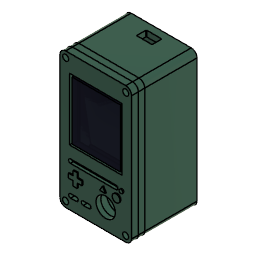
BMO (Autodesk Fusion 360 design; units mm, degrees)
Autodesk Fusion 360 part; units mm, degrees
note: some values were not read from the file. Chosen so that the rebuilt part matches the saved one: which bodies a step acts on; which face or edge a step refers to.
sketch "Sketch1" plane through (0, 0, 0) normal (0, 0, 1) x (1, 0, 0)
  line L0 (-25, -20) -> (2, -20)
  line L1 (2, -20) -> (2, 20)
  line L2 (2, 20) -> (-25, 20)
  line L3 (-25, 20) -> (-25, -20)
  dimension "d1" = 27
  dimension "d2" = 40
  constraint horizontal L0
  constraint vertical L1
  constraint horizontal L2
  constraint vertical L3
  measures "d1" distance of L0.start L0.end
  measures "d2" distance of L0.start L2.end
extrude "Extrude1" add sketch "Sketch1" along normal blind 2 makes body 1
sketch "Sketch2" plane through (0, 0, 2) normal (0, 0, 1) x (-1, 0, 0)
  line L0 (25, -20) -> (25, 20)
  line L1 (25, 20) -> (-2, 20)
  line L2 (-2, 20) -> (-2, -20)
  line L3 (-2, -20) -> (25, -20)
  line L4 (11.5, 20) -> (11.5, 16)
  line L5 (11.5, -20) -> (11.5, -15)
  line L6 (25, -15) -> (-2, -15)
  line L7 (-2, -15) -> (-2, 15)
  line L8 (25, 15) -> (25, -15)
  line L9 (25, 15) -> (-2, 15)
  dimension "d5" = 4
  dimension "d6" = 5
  constraint midpoint L1 L4.start
  constraint perpendicular L1 L4
  constraint midpoint L3 L5.start
  constraint perpendicular L3 L5
  constraint coincident L0 L6.start
  constraint coincident L2 L6.end
  constraint perpendicular L2 L6
  constraint coincident L2 L7.end
  constraint perpendicular L1 L7
  constraint coincident L0 L8.start
  constraint perpendicular L7 L9
  measures "d5" distance of L4.start L4.end
  measures "d6" distance of L5.start L5.end
extrude "Extrude2" add sketch "Sketch2" along normal blind 3 contours L0 L2 L6 L7 L8 L9 bodies 1
sketch "Sketch3" plane through (0, 0, 5) normal (0, 0, 1) x (-1, 0, 0)
  line L0 (25, -15) -> (25, 15)
  line L1 (25, 15) -> (-2, 15)
  line L2 (-2, 15) -> (-2, -15)
  line L3 (-2, -15) -> (25, -15)
  line L4 (-1, 15) -> (-1, -15)
  line L5 (24, -15) -> (24, 15)
  dimension "d9" = -1
  dimension "d10" = -1
extrude "Extrude3" cut sketch "Sketch3" against normal up to surface (3 mm away) contours L1 L2 L3 L4 bodies 1
extrude "Extrude4" cut sketch "Sketch3" against normal up to surface (3 mm away) contours L0 L1 L3 L5 bodies 1
sketch "Sketch4" plane through (0, 0, 0) normal (0, 0, 1) x (1, 0, 0)
  line L0 (-5, -8) -> (22, -8)
  line L1 (22, -8) -> (22, 22)
  line L2 (22, 22) -> (-5, 22)
  line L3 (-5, 22) -> (-5, -8)
  line L4 (27, -13) -> (27, 27)
  line L5 (27, 27) -> (-10, 27)
  line L6 (-10, 27) -> (-10, -13)
  line L7 (-5, -13) -> (22, -13)
  line L8 (-10, -13) -> (-10, -38)
  line L9 (27, -13) -> (27, -38)
  line L10 (-10, -38) -> (-5, -38)
  line L11 (27, -38) -> (22, -38)
  line L12 (-5, -38) -> (-5, -13)
  line L13 (22, -38) -> (22, -13)
  dimension "d15" = 27
  dimension "d16" = 30
  dimension "d18" = 25
  dimension "d19" = 25
  dimension "d20" = 5
  dimension "d21" = 5
  constraint horizontal L0
  constraint vertical L1
  constraint horizontal L2
  constraint vertical L3
  constraint perpendicular L7 L8
  constraint perpendicular L7 L9
  constraint perpendicular L8 L10
  constraint perpendicular L9 L11
  constraint perpendicular L7 L12
  constraint perpendicular L7 L13
  measures "d15" distance of L0.start L0.end
  measures "d16" distance of L0.start L2.end
  measures "d18" distance of L6.end L8.end
  measures "d19" distance of L4.start L9.end
  measures "d20" distance of L8.end L10.end
  measures "d21" distance of L9.end L11.end
extrude "Extrude5" add sketch "Sketch4" along normal blind 5 separate body makes body 2
move_body "Move1" bodies 2 to x (1, 0, 0) y (0, 1, 0) z (0, 0, 1) at (-20, -7, -1)
extrude "Extrude6" cut 1 faces at (-7, 15, 2.3333) along direction (0, 1, 0) blind 1 on bodies 2 bodies 2
extrude "Extrude7" cut 1 faces at (-16, -15, 2.3333) along direction (0, -1, 0) blind 1 on bodies 2 bodies 2
sketch "Sketch5" plane through (0, -20, 0) normal (0, -1, 0) x (1, 0, 0)
  line L0 (-25, -1) -> (2, -1)
  line L1 (2, -1) -> (2, 4)
  line L2 (2, 4) -> (-25, 4)
  line L3 (-25, 4) -> (-25, -1)
  line L4 (-11.5, 0.2) -> (2, 0.2)
  line L5 (-11.5, 0.2) -> (-25, 0.2)
  line L6 (-25, 0.2) -> (-25, 1.4)
  line L7 (-25, 1.4) -> (2, 1.5)
  line L8 (2, 0.2) -> (2, 1.5)
  dimension "d29" = 1.2
  constraint coincident L1 L4.end
  constraint perpendicular L1 L4
  constraint coincident L3 L5.end
  constraint perpendicular L3 L5
  constraint perpendicular L5 L6
  constraint midpoint L1 L7.end
  measures "d29" distance of L5.end L6.end
extrude "Extrude8" cut sketch "Sketch5" against normal blind 42 contours L1 L3 L4 L5 L6 L7 L8 bodies 2
extrude "Extrude9" add 1 faces at (5.3333, -13.6667, 4) along direction (0, 0, 1) blind 2 on bodies 2 bodies 2
sketch "Sketch6" plane through (0, 20, 0) normal (0, 1, 0) x (-1, 0, 0)
  line L0 (-2, 0.2) -> (-2, 1.5)
  line L1 (-2, 1.5) -> (25, 1.4)
  line L2 (25, 1.4) -> (25, 0.2)
  line L3 (25, 0.2) -> (-2, 0.2)
  line L4 (-7, -1) -> (30, -1)
  line L5 (30, -1) -> (30, 6)
  line L6 (30, 6) -> (-7, 6)
  line L7 (-7, 6) -> (-7, -1)
  line L8 (-2, 0) -> (-2.5, 0)
  line L9 (-2.5, 2) -> (-2, 2)
  line L10 (25, 2) -> (25.5, 2)
  line L11 (25.5, 0) -> (-2, 0)
  line L12 (-2, 2) -> (-1, 2)
  line L13 (-1, 2) -> (-1, 5.2)
  line L14 (25, 2) -> (24, 2)
  line L15 (24, 2) -> (24, 5.2)
  line L16 (24, 5.2) -> (-1, 5.2)
  line L17 (25.5, 2) -> (25.5, 0)
  line L18 (-2.5, 0) -> (-2.5, 2)
  dimension "d36" = 1
  dimension "d38" = 1
  dimension "d39" = 3.2
  constraint perpendicular L0 L8
  constraint perpendicular L2 L10
  constraint perpendicular L13 L16
  measures "d36" distance of L9.end L12.end
  measures "d38" distance of L10.start L14.end
  measures "d39" distance of L14.end L15.end
extrude "Extrude10" cut sketch "Sketch6" against normal blind 40.5 contours L8 L9 L10 L11 L12 L13 L14 L15 L16 L17 L18 bodies 2
move_body "Move2" bodies 2 to x (1, 0, 0) y (0, 0, 1) z (0, -1, 0) at (0, -42.5, 47.5)
sketch "Sketch7" plane through (0, 0, 0) normal (0, 0, 1) x (1, 0, 0)
  line L0 (2, 41) -> (-25, 41)
  line L1 (7, 46) -> (-30, 46)
  line L2 (7, 46) -> (7, -29)
  line L3 (2, 41) -> (2, -29)
  line L4 (-25, 41) -> (-25, -29)
  line L5 (-30, 46) -> (-30, -29)
  line L6 (7, -29) -> (2, -29)
  line L7 (-25, -29) -> (-30, -29)
  dimension "d58" = 75
  dimension "d59" = 70
  dimension "d60" = 70
  dimension "d61" = 75
  constraint perpendicular L1 L2
  constraint perpendicular L0 L3
  constraint perpendicular L0 L4
  constraint perpendicular L1 L5
  measures "d58" distance of L1.start L2.end
  measures "d59" distance of L0.start L3.end
  measures "d60" distance of L0.end L4.end
  measures "d61" distance of L1.end L5.end
extrude "Extrude11" add sketch "Sketch7" along normal blind 7 separate body makes body 3
move_body "Move3" bodies 3 to x (1, 0, 0) y (0, 1, 0) z (0, 0, 1) at (0, -12.5, 2.5)
move_body "Move6" bodies 2 to x (1, 0, 0) y (0, 0.866025, -0.5) z (0, 0.5, 0.866025) at (0, -6.2478, -21.317)
move_body "Move7" bodies 1 to x (1, 0, 0) y (0, 0.573576, 0.819152) z (0, -0.819152, 0.573576) at (0, -8.5285, 16.383)
move_body "Move8" bodies 1 to x (1, 0, 0) y (0, 1, 0) z (0, 0, 1) at (0, -9.3976, 23.6016)
move_body "Move9" bodies 1 to x (1, 0, 0) y (0, 0.996195, 0.087156) z (0, -0.087156, 0.996195) at (0, 1.9389, 2.7948)
extrude "Extrude12" add 1 faces at (1, -13.5501, 59.3017) along direction (-1, 0, 0) blind 25 on bodies 2 bodies 2
extrude "Extrude13" cut 1 faces at (-16, -11.7026, 58.235) along direction (0, -0.866025, 0.5) blind 0.2 on bodies 2 bodies 2
extrude "Extrude14" add 1 faces at (1, -31.4085, 26.5034) along direction (-1, 0, 0) blind 27 on bodies 2 bodies 2
move_body "Move10" bodies 2 to x (1, 0, 0) y (0, 0.5, -0.866025) z (0, 0.866025, 0.5) at (0, -24.884, -39.9042)
extrude "Extrude15" add 1 faces at (2, -35.8022, -0.2519) along direction (-1, 0, 0) blind 27 on bodies 2 bodies 2
split "Split3" by plane through (1, -14.9689, -0.4519) normal (0, 0, -1) bodies 2 makes body 4 at (-7, -34.3022, -3.6519)
extrude "Extrude16" add 1 faces at (-7, -14.9689, -2.9853) along direction (0, 1, 0) blind 32 on bodies 4 bodies 4
sketch "Sketch8" plane through (0, 0, -2.6519) normal (0, 0, 1) x (-1, 0, 0)
  line L0 (25.5, 19.4689) -> (-2.5, 19.4689)
  line L1 (-2.5, 19.4689) -> (-2.5, -21.0311)
  line L2 (-2.5, -21.0311) -> (25.5, -21.0311)
  line L3 (25.5, -21.0311) -> (25.5, 19.4689)
  line L4 (4, 14.4689) -> (19, 14.4689)
  line L5 (20, 15.4689) -> (20, 19.4689)
  line L6 (20, 19.4689) -> (3, 19.4689)
  line L7 (3, 19.4689) -> (3, 15.4689)
  arc A0 (3, 15.4689) -> (4, 14.4689) centre (4, 15.4689) ccw
  arc A1 (19, 14.4689) -> (20, 15.4689) centre (19, 15.4689) ccw
  dimension "d83" = 1
  constraint horizontal L4
  constraint vertical L5
  constraint horizontal L6
  constraint vertical L7
  constraint tangent L7 A0
  constraint tangent L4 A0
  constraint tangent L4 A1
  constraint tangent L5 A1
  constraint equal A0 A1
  measures "d83" radius of A0
extrude "Extrude17" cut sketch "Sketch8" against normal blind 2 contours L0 L4 L5 L6 L7 A0 A1 bodies 4
extrude "Extrude18" add 1 faces at (5.5, 21.0311, -2.2519) along direction (0, 1, 0) blind 5 on bodies 4 bodies 4
split "Split4" by plane through (1, 21.0311, -0.6519) normal (0, 1, 0) bodies 4 makes body 5 at (-5.3333, 24.3644, -3.6519)
extrude "Extrude19" add 1 faces at (2.5, 22.6978, -1.9186) along direction (-1, 0, 0) blind 28 on bodies 5 bodies 4 5
extrude "Extrude20" add 1 faces at (-6.8333, 21.0311, 2.0814) along direction (0, 1, 0) up to surface (5 mm away) on bodies 2 bodies 2
sketch "Sketch9" plane through (0, 0, 3.3481) normal (0, 0, 1) x (-1, 0, 0)
  line L0 (-2, -17.0311) -> (-2, 14.9689)
  line L1 (-2, 14.9689) -> (25, 14.9689)
  line L2 (25, 14.9689) -> (25, -17.0311)
  line L3 (25, -17.0311) -> (-2, -17.0311)
  line L4 (-7, 43.9689) -> (-7, -26.0311)
  line L5 (-7, -26.0311) -> (30, -26.0311)
  line L6 (30, -26.0311) -> (30, 43.9689)
  line L7 (30, 43.9689) -> (-7, 43.9689)
  line L8 (30, -26.0311) -> (27, -26.0311)
  line L9 (30, -26.0311) -> (30, -23.0311)
  circle A0 centre (27, -23) radius 1.55
  line L10 (30, -23.0311) -> (-7, -23)
  line L11 (-7, -26.0311) -> (-4, -26.0311)
  line L12 (-7, 43.9689) -> (-7, 40.9689)
  line L13 (-7, 40.9689) -> (30, 40.9689)
  line L14 (-4, -26.0311) -> (-4, 40.9689)
  dimension "d93" = 3
  dimension "d94" = 3
  dimension "d95" = 3.1
  dimension "d98" = 3
  dimension "d99" = 3
  constraint coincident L5.end L6.start
  constraint perpendicular L6 L8
  constraint perpendicular L8 L9
  constraint coincident L4 L10.end
  constraint coincident L4.end L5.start
  constraint perpendicular L4 L11
  constraint coincident L4.start L7.end
  constraint perpendicular L7 L12
  constraint coincident L6 L13.end
  constraint perpendicular L6 L13
  constraint coincident L13 L14.end
  constraint perpendicular L13 L14
  measures "d93" distance of L5.end L8.end
  measures "d94" distance of L5.end L9.end
  measures "d95" diameter of A0
  measures "d98" distance of L4.end L11.end
  measures "d99" distance of L4.start L12.end
extrude "Extrude21" cut sketch "Sketch9" against normal blind 11 contours A0 L10 | A0 L10 bodies 2 4
pattern_linear "R-Pattern1" count 2 spacing 31 along (1, -0.00084, 0) count 2 spacing 64 along (-0.00084, -1, 0) of "Extrude21"
extrude "Extrude22" cut 1 faces at (-16.2025, -33.2495, -0.4519) along direction (0, 0, -1) blind 0.9 on bodies 4 bodies 4
move_body "Move11" bodies 4 to x (1, 0, 0) y (0, 1, 0) z (0, 0, 1) at (0, 0, 0.9)
extrude "Extrude23" cut 1 faces at (-16.0359, -31.6288, 3.3481) along direction (0, 0, -1) blind 0.3 on bodies 2 bodies 2
move_body "Move12" bodies 2 4 to x (1, 0, 0) y (0, 0, 1) z (0, -1, 0) at (0, -44.4208, 43.517)
sketch "Sketch10" plane through (0, 0, 0) normal (0, 0, 1) x (1, 0, 0)
  line L0 (-8, -10) -> (22, -10)
  line L1 (22, -10) -> (22, 45)
  line L2 (22, 45) -> (-8, 45)
  line L3 (-8, 45) -> (-8, -10)
  dimension "d108" = 30
  dimension "d109" = 55
  constraint horizontal L0
  constraint vertical L1
  constraint horizontal L2
  constraint vertical L3
  measures "d108" distance of L0.start L0.end
  measures "d109" distance of L0.start L2.end
extrude "Extrude24" add sketch "Sketch10" along normal blind 5 separate body makes body 6
move_body "Move13" bodies 6 to x (1, 0, 0) y (0, 0, 1) z (0, -1, 0) at (0, -5, 15)
move_body "Move14" bodies 6 to x (1, 0, 0) y (0, 1, 0) z (0, 0, 1) at (-19.0538, -31.6689, -2.483)
move_body "Move15" bodies 6 to x (1, 0, 0) y (0, 1, 0) z (0, 0, 1) at (0, 11, 0)
move_body "Move16" bodies 1 to x (1, 0, 0) y (0, 0.866025, 0.5) z (0, -0.5, 0.866025) at (0, 7.6876, 18.7981)
move_body "Move17" bodies 1 to x (1, 0, 0) y (0, 1, 0) z (0, 0, 1) at (-0.5, -13.0199, -0.6113)
extrude "Extrude25" cut 1 faces at (-9, -42.6689, 52.7147) along direction (0, 1, 0) blind 0.5 on bodies 4 bodies 4
move_body "Move18" bodies 1 to x (1, 0, 0) y (0, 1, 0) z (0, 0, 1) at (0, -5, 0)
move_body "Move19" bodies 1 to x (1, 0, 0) y (0, 1, 0) z (0, 0, 1) at (1, 5.5, 0)
move_body "Move20" bodies 1 to x (1, 0, 0) y (0, 1, 0) z (0, 0, 1) at (-0.5, 0, 0)
extrude "Extrude26" add 1 faces at (-14, -41.6689, 53.2108) along direction (0, 1, 0) blind 1 on bodies 4 bodies 4
move_body "Move21" bodies 6 to x (1, 0, 0) y (0, 1, 0) z (0, 0, 1) at (0, 0, 7)
sketch "Sketch11" plane through (0, 0, 0) normal (0, 0, 1) x (1, 0, 0)
  line L0 (5, -14) -> (-32, -14)
  line L1 (-32, -14) -> (-32, -44)
  line L2 (-32, -44) -> (5, -44)
  line L3 (5, -44) -> (5, -14)
  line L4 (-29, -17) -> (-29, -41)
  line L5 (-29, -41) -> (2, -41)
  line L6 (2, -41) -> (2, -17)
  line L7 (2, -17) -> (-29, -17)
  dimension "d117" = 37
  dimension "d118" = 30
  dimension "d119" = -3
  constraint horizontal L0
  constraint vertical L1
  constraint horizontal L2
  constraint vertical L3
  measures "d117" distance of L0.start L0.end
  measures "d118" distance of L0.start L2.end
extrude "Extrude27" add sketch "Sketch11" along normal blind 70 separate body makes body 7
split "Split5" by plane through (-29, -41, 0) normal (0, 1, 0) bodies 7 makes body 8 at (-7.3333, -14, 23.3333)
delete_body "RemoveBody5" bodies 7
sketch "Sketch12" plane through (0, -17, 0) normal (0, -1, 0) x (1, 0, 0)
  line L0 (-29, 0) -> (2, 0)
  line L1 (2, 0) -> (2, 70)
  line L2 (2, 70) -> (-29, 70)
  line L3 (-29, 70) -> (-29, 0)
  line L4 (-13.5, 70) -> (-13.5, 67)
  line L5 (-13.5, 67) -> (-11.4928, 67)
  line L6 (-11.4928, 67) -> (-13.5, 67)
  line L7 (-13.5, 67) -> (-13.5, 70)
  line L8 (-13.5, 70) -> (-11.4928, 70)
  line L9 (-11.4928, 70) -> (-11.4928, 67)
  dimension "d122" = 3
  constraint midpoint L2 L4.start
  constraint perpendicular L2 L4
  constraint perpendicular L4 L5
  constraint horizontal L6
  constraint vertical L7
  constraint horizontal L8
  constraint vertical L9
  measures "d122" distance of L4.start L4.end
extrude "Extrude28" add sketch "Sketch12" along normal up to surface (24 mm away) contours L2 L4 L5 L6 L7 L8 L9 bodies 8
extrude "Extrude29" add 1 faces at (-13.5, -33, 69) along direction (-1, 0, 0) blind 16 on bodies 8 bodies 8
extrude "Extrude30" add 1 faces at (-11.4928, -33, 69) along direction (1, 0, 0) blind 14 on bodies 8 bodies 8
move_body "Move22" bodies 4 to x (1, 0, 0) y (0, 1, 0) z (0, 0, 1) at (-2, -0.3311, 0.4519)
move_body "Move23" bodies 2 to x (1, 0, 0) y (0, 1, 0) z (0, 0, 1) at (-2, -0.3311, 0.4519)
sketch "Sketch13" plane through (0, -17, 0) normal (0, -1, 0) x (1, 0, 0)
  line L0 (2, 67) -> (-29, 67)
  line L1 (-29, 67) -> (-29, 0)
  line L2 (-29, 0) -> (2, 0)
  line L3 (2, 0) -> (2, 67)
  line L4 (-15, 0) -> (-13, 0)
  line L5 (-13, 0) -> (-13, 3)
  line L6 (-13, 3) -> (-15, 3)
  line L7 (-15, 3) -> (-15, 0)
  dimension "d129" = 3
  constraint horizontal L4
  constraint vertical L5
  constraint horizontal L6
  constraint vertical L7
  constraint coincident L2 L4.start
  measures "d129" distance of L4.start L6.end
extrude "Extrude31" add sketch "Sketch13" along normal up to surface (24 mm away) contours L2 L4 L5 L6 L7 bodies 8
extrude "Extrude32" add 1 faces at (-13, -33, 1) along direction (1, 0, 0) blind 16 on bodies 8 bodies 8
extrude "Extrude33" add 1 faces at (-15, -33, 2) along direction (-1, 0, 0) blind 15 on bodies 8 bodies 8
chamfer "Chamfer1" distance 4 angle 45 4 edges at (-29, -29, 3) (-29, -29, 67) (2, -29, 3) (2, -29, 67) on bodies 8
move_body "Move24" bodies 6 to x (1, 0, 0) y (0, 1, 0) z (0, 0, 1) at (-1.5, 0, -2)
move_body "Move25" bodies 1 to x (1, 0, 0) y (0, 1, 0) z (0, 0, 1) at (-2.5, -0.1311, 0.4519)
move_body "Move26" bodies 1 to x (1, 0, 0) y (0, 1, 0) z (0, 0, 1) at (0, -10, 0)
move_body "Move27" bodies 1 to x (1, 0, 0) y (0, 1, 0) z (0, 0, 1) at (0, 9.8, 0)
move_body "Move28" bodies 1 to x (1, 0, 0) y (0, 1, 0) z (0, 0, 1) at (0.5, 0, 0.2)
delete_body "RemoveBody6" bodies 3
sketch "Sketch14" plane through (0, -44.3, 0) normal (0, 1, 0) x (-1, 0, 0)
  circle A0 centre (-1.9462, 2.9429) radius 1.55
  circle A1 centre (29.0538, 2.9689) radius 1.55
  circle A2 centre (-2, 66.9429) radius 1.55
  circle A3 centre (29, 66.9689) radius 1.55
  line L0 (-5, 70) -> (-5, 0)
  line L1 (-5, 0) -> (32, 0)
  line L2 (32, 0) -> (32, 70)
  line L3 (32, 70) -> (-5, 70)
  line L4 (27, 29) -> (0, 29)
  line L5 (0, 29) -> (0, 61)
  line L6 (0, 61) -> (27, 61)
  line L7 (27, 61) -> (27, 29)
  circle A4 centre (8.3739, 10.4932) radius 5
  circle A5 centre (2.5169, 17.6782) radius 2
  line L8 (8, 17) -> (11, 17)
  line L9 (11, 17) -> (9.5, 19.5981)
  line L10 (9.5, 19.5981) -> (8, 17)
  circle A6 centre (0, 22) radius 1
  line L11 (3, 23) -> (26.569, 23)
  line L12 (3, 21) -> (26.569, 21)
  arc A7 (3, 23) -> (3, 21) centre (3, 22) ccw
  arc A8 (26.569, 21) -> (26.569, 23) centre (26.569, 22) ccw
  line L13 (22.5236, 19.0194) -> (24.7236, 19.0194)
  line L14 (24.7236, 12.0194) -> (22.5236, 12.0194)
  line L15 (22.5236, 16.6194) -> (20.1236, 16.6194)
  line L16 (27.1236, 16.6194) -> (27.1236, 14.4194)
  line L17 (20.1236, 14.4194) -> (20.1236, 16.6194)
  line L18 (22.5236, 12.0194) -> (22.5236, 14.4194)
  line L19 (22.5236, 16.6194) -> (22.5236, 19.0194)
  line L20 (27.1236, 14.4194) -> (24.7236, 14.4194)
  line L21 (22.5236, 14.4194) -> (20.1236, 14.4194)
  line L22 (24.7236, 19.0194) -> (24.7236, 16.6194)
  line L23 (24.7236, 14.4194) -> (24.7236, 12.0194)
  line L24 (20.1236, 16.6194) -> (22.5236, 16.6194)
  line L25 (24.7236, 16.6194) -> (27.1236, 16.6194)
  line L26 (16.933, 7.5163) -> (19.9463, 7.5163)
  line L27 (16.963, 5.5165) -> (19.9462, 5.5163)
  line L28 (23.3591, 7.5092) -> (26.4396, 7.5298)
  arc A9 (19.9462, 5.5163) -> (19.9463, 7.5163) centre (19.9463, 6.5163) ccw
  arc A10 (16.933, 7.5163) -> (16.963, 5.5165) centre (16.9463, 6.5164) ccw
  line L29 (23.489, 5.514) -> (26.4516, 5.5298)
  arc A11 (23.5201, 7.5103) -> (23.489, 5.514) centre (23.4463, 6.513) ccw
  arc A12 (26.4516, 5.5298) -> (26.4396, 7.5298) centre (26.4462, 6.5298) ccw
  circle A13 centre (8.3739, 10.4932) radius 6.5
  dimension "d137" = 10
  dimension "d138" = 4
  dimension "d139" = 60
  dimension "d140" = 3
  dimension "d141" = 2
  dimension "d142" = 2.2
  dimension "d143" = 7
  dimension "d147" = 7
  dimension "d148" = 2.2
  dimension "d151" = 2
  dimension "d152" = 3
  dimension "d153" = 2
  dimension "d154" = 3.5
  dimension "d155" = 2
  dimension "d156" = 3
  dimension "d157" = 2
  dimension "d170" = 13
  constraint horizontal L8
  constraint tangent L11 A8
  constraint tangent L12 A8
  constraint horizontal L13
  constraint vertical L22
  constraint horizontal L14
  constraint vertical L18
  constraint perpendicular L15 L18
  constraint horizontal L24
  constraint vertical L16
  constraint horizontal L20
  constraint vertical L17
  constraint coincident L18.end L20
  constraint collinear L18 L19
  constraint coincident L20.end L22
  constraint collinear L20 L21
  constraint coincident L22.end L24
  constraint collinear L22 L23
  constraint collinear L24 L25
  constraint tangent L26 A9
  constraint horizontal L26
  constraint tangent L27 A9
  constraint coincident L28.start A11
  constraint tangent L28 A12
  constraint tangent L29 A12
  constraint coincident L28 A11.start
  constraint concentric A4 A13
  measures "d137" diameter of A4
  measures "d138" diameter of A5
  measures "d139" angle of L8 L9
  measures "d140" distance of L8.end L9.end
  measures "d141" diameter of A8
  measures "d142" distance of L13.start L13.end
  measures "d143" distance of L13.start L14.end
  measures "d147" distance of L15.end L16.start
  measures "d148" distance of L15.end L17.start
  measures "d151" diameter of A10
  measures "d152" distance of A10.centre A9.centre
  measures "d153" diameter of A9
  measures "d154" distance of A9.centre A11.centre
  measures "d155" diameter of A11
  measures "d156" distance of A11.centre A12.centre
  measures "d157" diameter of A12
  measures "d170" diameter of A13
extrude "Extrude34" cut sketch "Sketch14" against normal blind 13 contours A4 bodies 2
extrude "Extrude35" add sketch "Sketch14" against normal blind 4 contours A5 bodies 2
extrude "Extrude36" add sketch "Sketch14" against normal blind 4 contours L8 L9 L10 bodies 2
extrude "Extrude37" add sketch "Sketch14" against normal blind 4 contours A6 | L13 L14 L15 L16 L17 L18 L19 L20 L21 L22 L23 L24 L25 | L26 L27 A9 A10 | L28 L29 A11 A12 bodies 2
extrude "Extrude38" add sketch "Sketch14" against normal blind 5 contours L11 L12 A7 A8 bodies 2
extrude "Extrude39" cut 1 faces at (-10.8563, -49.3, 22.3333) along direction (0, 1, 0) blind 3 on bodies 2 bodies 2
extrude "Extrude40" cut sketch "Sketch14" against normal blind 1 contours A13 bodies 2
extrude "Extrude41" cut sketch "Sketch14" along normal blind 1 contours A4 bodies 4
extrude "Extrude42" cut sketch "Sketch14" along normal blind 9 contours A4 | A13 bodies 4
sketch "Sketch15" plane through (0, -41, 0) normal (0, 1, 0) x (-1, 0, 0)
  circle A0 centre (8.3739, 10.4932) radius 6.5
  circle A1 centre (-1.9462, 2.9429) radius 1.55
  circle A2 centre (29.0538, 2.9689) radius 1.55
  circle A3 centre (-2, 66.9429) radius 1.55
  circle A4 centre (29, 66.9689) radius 1.55
  line L0 (-5, 70) -> (-5, 0)
  line L1 (-5, 0) -> (32, 0)
  line L2 (32, 0) -> (32, 70)
  line L3 (32, 70) -> (-5, 70)
  line L4 (22, 28.5) -> (22, 24.5)
  line L5 (22, 24.5) -> (5, 24.5)
  line L6 (5, 24.5) -> (5, 28.5)
  arc A5 (6, 29.5) -> (5, 28.5) centre (6, 28.5) ccw
  line L7 (6, 29.5) -> (21, 29.5)
  arc A6 (22, 28.5) -> (21, 29.5) centre (21, 28.5) ccw
  circle A7 centre (8.3739, 10.4932) radius 6.5
  line L8 (3.3739, 15.4932, 3.2) -> (13.3739, 15.4932, 3.2)
  line L9 (13.3739, 15.4932, 3.2) -> (13.3739, 5.4932, 3.2)
  line L10 (13.3739, 5.4932, 3.2) -> (3.3739, 5.4932, 3.2)
  line L11 (3.3739, 5.4932, 3.2) -> (3.3739, 15.4932, 3.2)
  dimension "d180" = 10
  dimension "d181" = 10
  constraint concentric A0 A7
extrude "Extrude43" cut 2 faces at (-24.4292, -48.3, 6.851) (-17.9474, -48.3, 6.8497) along direction (0, 1, 0) blind 2.5 on bodies 2 bodies 2
extrude "Extrude52" cut sketch "Sketch15" along normal blind 25 contours A1 | A2 | A3 | A4 bodies 8
extrude "Extrude53" add 1 faces at (-18.5538, -30.6689, 44.1837) along direction (0, -1, 0) blind 5 on bodies 6 bodies 6
sketch "Sketch18" plane through (0, 0, 7.517) normal (0, 0, -1) x (1, 0, 0)
  line L0 (-28.5538, 25.6689) -> (1.4462, 25.6689)
  line L1 (1.4462, 25.6689) -> (1.4462, 35.6689)
  line L2 (1.4462, 35.6689) -> (-28.5538, 35.6689)
  line L3 (-28.5538, 35.6689) -> (-28.5538, 25.6689)
  line L4 (-13.5538, 25.6689) -> (-22.0538, 25.6689)
  line L5 (-13.5538, 25.6689) -> (-5.0538, 25.6689)
  line L6 (-5.0538, 25.6689) -> (-22.0538, 25.6689)
  line L7 (-22.0538, 25.6689) -> (-22.0538, 35.6689)
  line L8 (-22.0538, 35.6689) -> (-5.0538, 35.6689)
  line L9 (-5.0538, 35.6689) -> (-5.0538, 25.6689)
  dimension "d208" = 8.5
  dimension "d209" = 8.5
  constraint midpoint L0 L4.start
  constraint parallel L0 L4
  constraint parallel L0 L5
  constraint horizontal L6
  constraint vertical L7
  constraint horizontal L8
  constraint vertical L9
  constraint coincident L2 L7.end
  measures "d208" distance of L4.start L4.end
  measures "d209" distance of L4.start L5.end
extrude "Extrude54" cut sketch "Sketch18" against normal blind 5 contours L0 L2 L3 L7 | L0 L1 L2 L9 bodies 6
sketch "Sketch19" plane through (0, 0, 62.517) normal (0, 0, 1) x (-1, 0, 0)
  line L0 (-1.4462, 25.6689) -> (28.5538, 25.6689)
  line L1 (28.5538, 25.6689) -> (28.5538, 35.6689)
  line L2 (28.5538, 35.6689) -> (-1.4462, 35.6689)
  line L3 (-1.4462, 35.6689) -> (-1.4462, 25.6689)
  line L4 (13.5538, 25.6689) -> (9.5538, 25.6689)
  line L5 (9.5538, 25.6689) -> (17.5538, 25.6689)
  line L6 (17.5538, 25.6689) -> (17.5538, 30.6689)
  line L7 (17.5538, 30.6689) -> (9.5538, 30.6689)
  line L8 (9.5538, 30.6689) -> (9.5538, 25.6689)
  dimension "d214" = 4
  constraint midpoint L0 L4.start
  constraint horizontal L5
  constraint vertical L6
  constraint horizontal L7
  constraint vertical L8
  measures "d214" distance of L4.start L4.end
extrude "Extrude55" add sketch "Sketch19" along normal blind 0.1 contours L0 L4 L5 L6 L7 L8 bodies 6
sketch "Sketch20" plane through (0, 0, 62.517) normal (0, 0, 1) x (-1, 0, 0)
  line L0 (17.5538, 30.6689) -> (17.5538, 25.6689)
  line L1 (17.5538, 25.6689) -> (28.5538, 25.6689)
  line L2 (28.5538, 25.6689) -> (28.5538, 35.6689)
  line L3 (28.5538, 35.6689) -> (-1.4462, 35.6689)
  line L4 (-1.4462, 35.6689) -> (-1.4462, 25.6689)
  line L5 (-1.4462, 25.6689) -> (9.5538, 25.6689)
  line L6 (9.5538, 25.6689) -> (9.5538, 30.6689)
  line L7 (9.5538, 30.6689) -> (17.5538, 30.6689)
  line L8 (17.5538, 30.6689) -> (24.5538, 30.6689)
  line L9 (9.5538, 30.6689) -> (2.5538, 30.6689)
  line L10 (24.5538, 30.6689) -> (2.5538, 30.6689)
  line L11 (2.5538, 30.6689) -> (2.5538, 35.6689)
  line L12 (2.5538, 35.6689) -> (24.5538, 35.6689)
  line L13 (24.5538, 35.6689) -> (24.5538, 30.6689)
  dimension "d217" = 7
  dimension "d218" = 7
  constraint coincident L0.start L7.end
  constraint perpendicular L2 L8
  constraint coincident L6.end L7.start
  constraint perpendicular L6 L9
  constraint horizontal L10
  constraint vertical L11
  constraint horizontal L12
  constraint vertical L13
  constraint coincident L3 L11.end
  measures "d217" distance of L0.start L8.end
  measures "d218" distance of L6.end L9.end
extrude "Extrude56" cut sketch "Sketch20" against normal up to surface (55 mm away) contours L3 L7 L8 L9 L10 L11 L12 L13 bodies 6
move_body "Move31" bodies 6 to x (1, 0, 0) y (0, 1, 0) z (0, 0, 1) at (0, 8, 8)
move_body "Move32" bodies 6 to x (1, 0, 0) y (0, 1, 0) z (0, 0, 1) at (0, 0, -4)
extrude "Extrude57" cut 1 faces at (-12.2204, -19.3356, 66.617) along direction (0, 0, 1) blind 9 on bodies 6 bodies 8
fillet "Fillet1" radius 0.25 4 edges at (-17.5538, -17.6689, 68.5) (-9.5538, -17.6689, 68.5) (-17.5538, -22.6689, 68.5) (-9.5538, -22.6689, 68.5) on bodies 8
move_body "Move33" bodies 6 to x (1, 0, 0) y (0, 1, 0) z (0, 0, 1) at (0, 0, -4)
sketch "Sketch21" plane through (0, -17, 0) normal (0, -1, 0) x (1, 0, 0)
  line L0 (2, 63) -> (-2, 67)
  line L1 (-2, 67) -> (-25, 67)
  line L2 (-25, 67) -> (-29, 63)
  line L3 (-29, 63) -> (-29, 7)
  line L4 (-29, 7) -> (-25, 3)
  line L5 (-25, 3) -> (-2, 3)
  line L6 (-2, 3) -> (2, 7)
  line L7 (2, 7) -> (2, 63)
  line L8 (-29, 12.5) -> (-23.5, 12.5)
  line L9 (-23.5, 12.5) -> (-23.5, 10.5)
  line L10 (-23.5, 10.5) -> (-29, 10.5)
  line L11 (-29, 10.5) -> (-29, 12.5)
  line L12 (2, 12.5) -> (-3.5, 12.5)
  line L13 (-3.5, 12.5) -> (-3.5, 10.5)
  line L14 (-3.5, 10.5) -> (2, 10.5)
  line L15 (2, 10.5) -> (2, 12.5)
  constraint horizontal L8
  constraint vertical L9
  constraint horizontal L10
  constraint vertical L11
  constraint coincident L3 L8.start
  constraint horizontal L12
  constraint vertical L13
  constraint horizontal L14
  constraint vertical L15
  constraint coincident L7 L12.start
extrude "Extrude58" add sketch "Sketch21" along normal blind 24 contours L7 L12 L13 L14 L15 | L3 L8 L9 L10 L11 bodies 8
sketch "Sketch15 (curves 3.2 mm off its plane)" plane through (0, -37.8, 0) normal (0, 1, 0) x (-1, 0, 0)
  line L0 (3.3739, 15.4932) -> (13.3739, 15.4932)
  line L1 (13.3739, 15.4932) -> (13.3739, 5.4932)
  line L2 (13.3739, 5.4932) -> (3.3739, 5.4932)
  line L3 (3.3739, 5.4932) -> (3.3739, 15.4932)
extrude "Extrude59" add sketch "Sketch15 (curves 3.2 mm off its plane)" along normal blind 3 separate body makes body 9
combine "Combine4" operation add target body 8 tool bodies 9 keep tools
delete_body "RemoveBody7" bodies 9
extrude "Extrude60" add 1 faces at (-3.3739, -36.8, 7.1621) along direction (1, 0, 0) blind 5 on bodies 8 bodies 8
extrude "Extrude61" add 1 faces at (-13.3739, -36.8, 12.1599) along direction (-1, 0, 0) blind 16 on bodies 8 bodies 8
extrude "Extrude62" add 1 faces at (-3.3739, -36.8, 13.4977) along direction (1, 0, 0) blind 5 on bodies 8 bodies 8
extrude "Extrude63" add 1 faces at (1.6261, -36.8, 13.4977) along direction (1, 0, 0) blind 0.5 on bodies 8 bodies 8
extrude "Extrude64" add 1 faces at (1.6261, -36.8, 7.9174) along direction (1, 0, 0) blind 1 on bodies 8 bodies 8
fillet "Fillet2" radius 3 12 edges at (5, -46.05, 0) (5, -46.05, 70) (-32, -46.05, 70) (-32, -46.05, 0) (5, -42.65, 0) (5, -42.65, 70) (-32, -42.65, 70) (-32, -42.65, 0) (5, -27.5, 0) (5, -27.5, 70) (-32, -27.5, 70) (-32, -27.5, 0) on bodies 2 4 8
sketch "Sketch22" plane through (0, -41, 0) normal (0, -1, 0) x (1, 0, 0)
  arc A0 (-32, 3) -> (-29, 0) centre (-29, 3) ccw
  line L0 (-29, 0) -> (2, 0)
  arc A1 (2, 0) -> (5, 3) centre (2, 3) ccw
  line L1 (5, 3) -> (5, 67)
  arc A2 (5, 67) -> (2, 70) centre (2, 67) ccw
  line L2 (2, 70) -> (-29, 70)
  arc A3 (-29, 70) -> (-32, 67) centre (-29, 67) ccw
  line L3 (-32, 67) -> (-32, 3)
  line L4 (-25, 3) -> (-29, 7)
  line L5 (-29, 7) -> (-29, 10.5)
  line L6 (-29, 10.5) -> (-23.5, 10.5)
  line L7 (-23.5, 10.5) -> (-23.5, 12.5)
  line L8 (-23.5, 12.5) -> (-29, 12.5)
  line L9 (-29, 12.5) -> (-29, 63)
  line L10 (-29, 63) -> (-25, 67)
  line L11 (-25, 67) -> (-2, 67)
  line L12 (-2, 67) -> (2, 63)
  line L13 (2, 63) -> (2, 12.5)
  line L14 (2, 12.5) -> (-3.5, 12.5)
  line L15 (-3.5, 12.5) -> (-3.5, 10.5)
  line L16 (-3.5, 10.5) -> (2, 10.5)
  line L17 (2, 10.5) -> (2, 7)
  line L18 (2, 7) -> (-2, 3)
  line L19 (-2, 3) -> (-25, 3)
  circle A4 centre (1.9462, 2.9429) radius 1.55
  circle A5 centre (2, 66.9429) radius 1.55
  circle A6 centre (-29.0538, 2.9689) radius 1.55
  circle A7 centre (-29, 66.9689) radius 1.55
  line L20 (-3.5, 12.5) -> (2, 12.5)
  line L21 (2, 12.5) -> (2, 10.5)
  line L22 (2, 10.5) -> (-3.5, 10.5)
  line L23 (-3.5, 10.5) -> (-3.5, 12.5)
  line L24 (-23.5, 12.5) -> (-29, 12.5)
  line L25 (-29, 12.5) -> (-29, 10.5)
  line L26 (-29, 10.5) -> (-23.5, 10.5)
  line L27 (-23.5, 10.5) -> (-23.5, 12.5)
  line L28 (-29, 12.5) -> (-30.5, 12.5)
  line L29 (-30.5, 12.5) -> (-30.5, 10.5)
  line L30 (-30.5, 10.5) -> (-29, 10.5)
  line L31 (-29, 10.5) -> (-29, 12.5)
  line L32 (2, 12.5) -> (3.5, 12.5)
  line L33 (3.5, 12.5) -> (3.5, 10.5)
  line L34 (3.5, 10.5) -> (2, 10.5)
  line L35 (2, 10.5) -> (2, 12.5)
  constraint horizontal L20
  constraint vertical L21
  constraint horizontal L22
  constraint vertical L23
  constraint coincident L16.end L17.start
  constraint coincident L14.end L15.start
  constraint horizontal L24
  constraint vertical L25
  constraint horizontal L26
  constraint vertical L27
  constraint coincident L5.end L6.start
  constraint coincident L7.end L8.start
  constraint horizontal L28
  constraint vertical L29
  constraint horizontal L30
  constraint vertical L31
  constraint horizontal L32
  constraint vertical L33
  constraint horizontal L34
  constraint vertical L35
extrude "Extrude65" cut sketch "Sketch22" against normal up to surface (3.2 mm away) contours L6 L7 L8 L24 L25 L26 L27 L31 | L14 L15 L16 L20 L21 L22 L23 L35 bodies 8
extrude "Extrude66" cut sketch "Sketch22" against normal up to surface (24 mm away) contours L25 L28 L29 L30 L31 | L21 L32 L33 L34 L35 bodies 8
split "Split6" by plane through (2, -41, 0) normal (-1, 0, 0) bodies 8 makes body 10 at (-9.3333, -14, 45.6667)
split "Split7" by plane through (2, -17, 0) normal (0, -1, 0) bodies 10 makes body 11 at (-32, -25, 24.3333)
split "Split8" by plane through (-29, -17, 0) normal (1, 0, 0) bodies 11 makes body 12 at (-12.2679, -34.8896, 70) makes body 13 at (-8.3333, -25, 0)
split "Split9" by plane through (1.6261, -37.8, 6.6261) normal (0, -1, 0) bodies 13 makes body 14 at (-17.3333, -41, 1)
split "Split10" by plane through (-13.3739, -37.8, 5.4932) normal (0, 0, -1) bodies 13 makes body 15 at (-8.3333, -23.9333, 0)
split "Split11" by plane through (1.6261, -34.8, 6.6261) normal (0, 1, 0) bodies 13 makes body 16 at (0.9955, -28.8667, 5.9955) makes body 17 at (-27.9955, -28.8667, 5.9955) makes body 18 at (-25.3333, -22.9333, 10.5) makes body 19 at (-1.6667, -22.9333, 10.5)
combine "Combine5" operation add target body 18 tool bodies 13
combine "Combine6" operation add target body 19 tool bodies 18
extrude "Extrude67" cut 1 faces at (-18.6667, -37.8, 8.8311) along direction (0, -1, 0) blind 5 on bodies 19 bodies 14
combine "Combine7" operation add target body 10 tool bodies 16 15 11 12 14 17
combine "Combine8" operation add target body 10 tool bodies 8
sketch "Sketch23" plane through (-29, 0, 0) normal (-1, 0, 0) x (0, -1, 0)
  line L0 (34.8, 12.5) -> (17, 12.5)
  line L1 (17, 12.5) -> (17, 10.5)
  line L2 (17, 10.5) -> (34.8, 10.5)
  line L3 (34.8, 10.5) -> (34.8, 5.4932)
  line L4 (34.8, 5.4932) -> (37.8, 5.4932)
  line L5 (37.8, 5.4932) -> (37.8, 15.4932)
  line L6 (37.8, 15.4932) -> (34.8, 15.4932)
  line L7 (34.8, 15.4932) -> (34.8, 12.5)
  line L8 (17, 12.5) -> (37.8, 12.5)
  line L9 (37.8, 12.5) -> (37.8, 10.4932)
  line L10 (37.8, 10.4932) -> (17, 10.4932)
  line L11 (17, 10.4932) -> (17, 12.5)
  constraint horizontal L8
  constraint vertical L9
  constraint horizontal L10
  constraint vertical L11
  constraint midpoint L5 L9.end
  constraint coincident L0.end L1.start
extrude "Extrude68" add sketch "Sketch23" along normal blind 1.4 contours L0 L1 L2 L3 L5 L8 L9 L10 L11 bodies 19
extrude "Extrude69" cut 1 faces at (-28.1, -28.8667, 10.5) along direction (0, 0, 1) blind 0.2 on bodies 19 bodies 19
extrude "Extrude70" cut 1 faces at (-29.4667, -36.8, 10.4932) along direction (0, 0, 1) up to surface (0.2068 mm away) on bodies 19 bodies 19
sketch "Sketch24" plane through (2, 0, 0) normal (1, 0, 0) x (0, 1, 0)
  line L0 (-34.8, 10.5) -> (-17, 10.5)
  line L1 (-17, 10.5) -> (-17, 12.5)
  line L2 (-17, 12.5) -> (-34.8, 12.5)
  line L3 (-34.8, 12.5) -> (-34.8, 15.4932)
  line L4 (-34.8, 15.4932) -> (-37.8, 15.4932)
  line L5 (-37.8, 15.4932) -> (-37.8, 5.4932)
  line L6 (-37.8, 5.4932) -> (-34.8, 5.4932)
  line L7 (-34.8, 5.4932) -> (-34.8, 10.5)
  line L8 (-17, 12.5) -> (-37.8, 12.5)
  line L9 (-37.8, 12.5) -> (-37.8, 10.4932)
  line L10 (-37.8, 10.4932) -> (-17, 10.4932)
  line L11 (-17, 10.4932) -> (-17, 12.5)
  constraint horizontal L8
  constraint vertical L9
  constraint horizontal L10
  constraint vertical L11
  constraint midpoint L5 L9.end
  constraint coincident L1.end L2.start
extrude "Extrude71" add sketch "Sketch24" along normal blind 1.4 contours L0 L1 L2 L5 L7 L8 L9 L10 L11 bodies 19
extrude "Extrude72" cut 1 faces at (1.1, -28.8667, 10.5) along direction (0, 0, 1) blind 0.2 on bodies 19 bodies 19
extrude "Extrude73" cut 1 faces at (2.9333, -35.8, 10.4932) along direction (0, 0, 1) up to surface (0.2068 mm away) on bodies 19 bodies 19
extrude "Extrude74" cut 1 faces at (-18.6667, -35.8, 5.4932) along direction (0, 0, 1) blind 0.2 on bodies 19 bodies 19
extrude "Extrude75" cut 2 faces at (-29, -35.8, 7.2932) (-29, -36.8, 10.5621) along direction (1, 0, 0) blind 0.1 on bodies 19 bodies 19
extrude "Extrude76" cut 1 faces at (2, -35.8, 7.2932) along direction (-1, 0, 0) blind 0.1 on bodies 19 bodies 19
extrude "Extrude77" cut 1 faces at (2, -35.8, 14.4955) along direction (-1, 0, 0) blind 0.1 on bodies 19 bodies 19
extrude "Extrude78" cut 1 faces at (-29, -36.8, 13.4977) along direction (1, 0, 0) blind 0.1 on bodies 19 bodies 19
extrude "Extrude44" [suppressed]
extrude "Extrude45" [suppressed]
extrude "Extrude46" [suppressed]
move_body "Move29" [suppressed]
combine "Combine2" [suppressed]
extrude "Extrude47" [suppressed]
move_body "Move30" [suppressed]
combine "Combine3" [suppressed]
sketch "Sketch16" plane through (0, 21.3311, 0) normal (0, -1, 0) x (1, 0, 0)
  line L0 (1.4462, 9.517) -> (-28.5538, 9.517)
  line L1 (-28.5538, 9.517) -> (-28.5538, 4.517)
  line L2 (-28.5538, 4.517) -> (1.4462, 4.517)
  line L3 (1.4462, 4.517) -> (1.4462, 9.517)
  line L4 (-13.5538, 9.517) -> (-9.5538, 9.517)
  line L5 (-13.5538, 9.517) -> (-17.5538, 9.517)
  line L6 (-17.5538, 9.517) -> (-17.5538, 4.517)
  line L7 (-17.5538, 4.517) -> (-9.5538, 4.517)
  line L8 (-9.5538, 4.517) -> (-9.5538, 9.517)
  line L9 (-17.5538, 9.517) -> (-17.5538, 4.517)
  dimension "d192" = 4
  dimension "d193" = 4
  constraint coincident L2 L6.end
  constraint perpendicular L2 L6
  constraint horizontal L7
  constraint vertical L8
  constraint vertical L9
  measures "d192" distance of L4.start L4.end
  measures "d193" distance of L4.start L5.end
extrude "Extrude48" [suppressed]
extrude "Extrude49" [suppressed]
extrude "Extrude50" [suppressed]
chamfer "Chamfer2" [suppressed]
chamfer "Chamfer3" [suppressed]
sketch "Sketch17" plane through (0, -44.3, 0) normal (0, -1, 0) x (1, 0, 0)
  circle A0 centre (-8.3739, 10.4932) radius 6.5
  circle A1 centre (1.9462, 2.9429) radius 1.55
  circle A2 centre (-29.0538, 2.9689) radius 1.55
  circle A3 centre (2, 66.9429) radius 1.55
  circle A4 centre (-29, 66.9689) radius 1.55
  line L0 (0.5, 65) -> (0.5, 24.5)
  line L1 (0.5, 24.5) -> (-27.5, 24.5)
  line L2 (-27.5, 24.5) -> (-27.5, 65)
  line L3 (-27.5, 65) -> (0.5, 65)
  line L4 (5, 70) -> (-32, 70)
  line L5 (-32, 70) -> (-32, 0)
  line L6 (-32, 0) -> (5, 0)
  line L7 (5, 0) -> (5, 70)
  circle A5 centre (1.9462, 2.9429) radius 1.55
  circle A6 centre (-29.0538, 2.9689) radius 1.55
  circle A7 centre (2, 66.9429) radius 1.55
  circle A8 centre (-29, 66.9689) radius 1.55
  constraint concentric A1 A5
  constraint concentric A2 A6
  constraint concentric A3 A7
  constraint concentric A4 A8
extrude "Extrude51" [suppressed]
move_body "Move4" [suppressed]
move_body "Move5" [suppressed]
split "Split1" [suppressed]
delete_body "RemoveBody1" bodies 20
delete_body "RemoveBody2" bodies 21
split "Split2" [suppressed]
delete_body "RemoveBody3" bodies 22
delete_body "RemoveBody4" bodies 23
combine "Combine1" [suppressed]
named bodies: "ekran", "ekran ön kapak", "ana gövde iskelet", "ekran arka kapak", "ekran arka kapak (1)", "esp", "ana gövde iskelet", "ana gövde iskelet (1) (1)", "ana gövde iskelet (1) (1) (1)", "ana gövde iskelet (1) (1) (2)", "ana gövde iskelet (1) (1) (2) (1)", "ana gövde iskelet (1) (1) (2) (2)", "ana gövde iskelet (1) (1) (2) (3)", "ana gövde iskelet (1) (1) (2) (4)", "ana gövde iskelet (1) (1) (2) (5)", "oturak"
